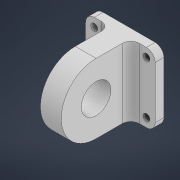
# Autodesk Inventor part: Hinge
Saved by Autodesk Inventor 2021 (Build 250183000, 183)
## iProperties
Created: 2021-01-30
Part Number: Hinge
Material: Generic
Document SubType Name: Modeling
Designer: PaisW
Density: 1 g/cm^3
Appearance: Default
Author: PaisW
Autodesk Inventor part; units mm, degrees
ref_plane "YZ Plane" through (0, 0, 0) normal (1, 0, 0) x (0, 1, 0)
ref_plane "XZ Plane" through (0, 0, 0) normal (0, 1, 0) x (-1, 0, 0)
ref_plane "XY Plane" through (0, 0, 0) normal (0, 0, 1) x (1, 0, 0)
sketch "Sketch5" plane through (0, 0, 0) normal (0, 0, 1) x (1, 0, 0)
  line L0 (-15, 15) -> (15, 15) construction
  line L1 (15, 15) -> (15, -15) construction
  line L2 (15, -15) -> (-15, -15) construction
  line L3 (-15, -15) -> (-15, 15) construction
  line L4 (-15, 15) -> (15, -15) construction
  line L5 (15, 15) -> (-15, -15) construction
  circle A0 centre (-15, 15) radius 2
  circle A1 centre (15, 15) radius 2
  circle A2 centre (15, -15) radius 2
  circle A3 centre (-15, -15) radius 2
  line L6 (-15, 20) -> (15, 20)
  line L7 (20, 15) -> (20, -15)
  line L8 (15, -20) -> (-15, -20)
  line L9 (-20, -15) -> (-20, 15)
  line L10 (-20, 20) -> (20, -20) construction
  line L11 (20, 20) -> (-20, -20) construction
  arc A4 (20, 15) -> (15, 20) centre (15, 15) ccw
  arc A5 (15, -20) -> (20, -15) centre (15, -15) ccw
  arc A6 (-20, -15) -> (-15, -20) centre (-15, -15) ccw
  arc A7 (-15, 20) -> (-20, 15) centre (-15, 15) ccw
  point P0 (0, 0)
  dimension "d16" = 4
  dimension "d17" = 30
  dimension "d18" = 40
  dimension "d20" = 5
  constraints: 24 end point, 9 point on line, 8 centre point, 8 point on circle, 8 tangent, 6 equal radius, 4 coincident, 4 midpoint, 4 parallel, 3 perpendicular, 2 horizontal
  measures "d16" diameter of A0
  measures "d17" distance of L2.end L0.start
  measures "d18" distance of L10.end L11.end
  measures "d20" radius of A4
extrude "Extrusion5" add sketch "Sketch5" along normal blind 5
sketch "Sketch6" plane through (0, 0, 5) normal (0, 0, 1) x (1, 0, 0)
  line L0 (-15, -20) -> (15, -20) projected
  line L1 (-6, 20) -> (6, 20)
  line L2 (6, 20) -> (6, -20)
  line L3 (6, -20) -> (-6, -20)
  line L4 (-6, -20) -> (-6, 20)
  line L5 (-6, 20) -> (6, -20) construction
  line L6 (6, 20) -> (-6, -20) construction
  point P0 (0, 0)
  dimension "d23" = 12
  constraints: 12 end point, 2 midpoint, 2 parallel, 1 horizontal, 1 perpendicular, 1 point on line
  measures "d23" distance of L1.start L1.end
extrude "Extrusion6" add sketch "Sketch6" along normal blind 40
fillet "Fillet2" radius 5 2 edges at (6, 0, 5) (-6, 0, 5)
sketch "Sketch7" plane through (6, -20, 45) normal (1, 0, 0) x (0, 0, -1)
  circle A0 centre (20, 20) radius 8.5
  circle A1 centre (20, 20) radius 20
  line L0 (0, 0) -> (0, 40) projected
  line L1 (40, 0) -> (40, 40) projected
  line L2 (35, 0) -> (0, 0) projected
  line L3 (20, 0) -> (0, 0)
  line L4 (0, 0) -> (0, 40)
  line L5 (0, 40) -> (20, 40)
  line L6 (35, 40) -> (0, 40) projected
  point P0 (45, 20)
  point P1 (0, 20)
  dimension "d27" = 17
  constraints: 6 end point, 3 tangent, 2 centre point, 2 point on circle, 2 point on line, 1 coincident, 1 collinear
  measures "d27" diameter of A0
extrude "Extrusion7" cut sketch "Sketch7" against normal blind 50 contours A0 | A1 L0 L5 | L2 L0 A1
sketch "Sketch1" plane through (0, 0, 0) normal (0, 1, 0) x (-1, 0, 0)
  line L0 (27.5, 22.5) -> (-27.5, 22.5)
  line L1 (-27.5, 22.5) -> (-27.5, -22.5)
  line L2 (-27.5, -22.5) -> (27.5, -22.5)
  line L3 (27.5, -22.5) -> (27.5, 22.5)
  point P0 (0, 0)
  point P1 (27.5, 0)
  point P2 (0, -22.5)
  dimension "d0" = 45
  dimension "d1" = 55
  constraints: 8 end point, 2 midpoint, 2 parallel, 1 horizontal, 1 horizontal alignment, 1 perpendicular, 1 vertical alignment
  measures "d0" distance of L2.end L0.start
  measures "d1" distance of L1.end L2.end
sketch "Sketch2" plane through (0, 10, 0) normal (0, 1, 0) x (1, 0, 0)
  line L0 (-27.5, 22.5) -> (-27.5, -22.5) projected
  line L1 (-27.5, -22.5) -> (27.5, -22.5) projected
  line L2 (-27.5, 22.5) -> (-19.5, 22.5)
  line L3 (-19.5, 22.5) -> (-19.5, -22.5)
  line L4 (-19.5, -22.5) -> (-27.5, -22.5)
  line L5 (-27.5, -22.5) -> (-27.5, 22.5)
  line L6 (27.5, -22.5) -> (27.5, 22.5) projected
  line L7 (27.5, 22.5) -> (19.5, 22.5)
  line L8 (19.5, 22.5) -> (19.5, -22.5)
  line L9 (19.5, -22.5) -> (27.5, -22.5)
  line L10 (27.5, -22.5) -> (27.5, 22.5)
  point P0 (0, 0)
  dimension "d4" = 8
  dimension "d5" = 8
  constraints: 16 end point, 4 parallel, 2 horizontal, 2 perpendicular, 2 point on line
  measures "d4" distance between parallel lines of L0 L3
  measures "d5" distance between parallel lines of L6 L8
sketch "Sketch4" plane through (0, 0, 0) normal (0, -1, 0) x (1, 0, 0)
  line L0 (15, 15) -> (-15, 15) construction
  line L1 (-15, 15) -> (-15, -15) construction
  line L2 (-15, -15) -> (15, -15) construction
  line L3 (15, -15) -> (15, 15) construction
  line L4 (15, 15) -> (-15, -15) construction
  line L5 (-15, 15) -> (15, -15) construction
  circle A0 centre (15, -15) radius 2
  circle A1 centre (-15, -15) radius 2
  circle A2 centre (-15, 15) radius 2
  circle A3 centre (15, 15) radius 2
  point P0 (0, 0)
  dimension "d12" = 30
  dimension "d13" = 4
  constraints: 12 end point, 4 centre point, 4 coincident, 3 equal radius, 2 midpoint, 2 parallel, 2 perpendicular, 1 horizontal
  measures "d12" distance of L0.end L1.end
  measures "d13" diameter of A0
sketch "Sketch3" plane through (27.5, 0, 22.5) normal (1, 0, 0) x (0, 0, -1)
  circle A0 centre (22.5, 25) radius 15
  line L0 (22.5, 25) -> (22.5, 47.5) construction
  line L1 (45, 47.5) -> (0, 47.5) projected
  line L2 (22.5, 25) -> (45, 25) construction
  line L3 (45, 0) -> (45, 47.5) projected
  point P0 (22.5, 0)
  dimension "d9" = 30
  constraints: 4 end point, 1 centre point, 1 horizontal, 1 midpoint, 1 perpendicular, 1 point on line, 1 vertical alignment
  measures "d9" diameter of A0
body "Solid1"
body "Solid2"
